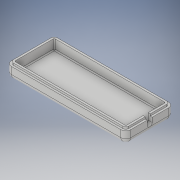
# Autodesk Inventor part: box_bottom
Saved by Autodesk Inventor 2017 (Build 210142000, 142)
## iProperties
Created: 2017-09-23
Part Number: box_bottom
Material: Generic
Document SubType Name: Modeling
Designer: Mitch
Density: 1 g/cm^3
Appearance: Default
Author: Mitch
Autodesk Inventor part; units mm, degrees
ref_plane "YZ Plane" through (0, 0, 0) normal (1, 0, 0) x (0, 1, 0)
ref_plane "XZ Plane" through (0, 0, 0) normal (0, 1, 0) x (-1, 0, 0)
ref_plane "XY Plane" through (0, 0, 0) normal (0, 0, 1) x (1, 0, 0)
sketch "Sketch1" plane through (0, 0, 0) normal (0, 1, 0) x (-1, 0, 0)
  line L0 (0, 0) -> (76.2, 0)
  line L1 (76.2, 0) -> (76.2, -30.48)
  line L2 (76.2, -30.48) -> (0, -30.48)
  line L3 (0, -30.48) -> (0, 0)
  dimension "d0" = 76.2
  dimension "d1" = 30.48
  constraints: 8 end point, 2 parallel, 1 horizontal, 1 perpendicular
  measures "d0" distance of L1.end L2.end
  measures "d1" distance of L0.end L1.end
extrude "Extrusion1" add sketch "Sketch1" along normal blind 8.89
fillet "Fillet1" radius 3.175 8 edges at (0, 4.445, 0) (0, 4.445, -30.48) (0, 0, -15.24) (-38.1, 0, 0) (-76.2, 4.445, 0) (-76.2, 0, -15.24) (-76.2, 4.445, -30.48) (-38.1, 0, -30.48)
shell "Shell1" thickness 2.54 removed faces 1 at (-26.4583, 8.89, -20.32)
sketch "Sketch2" plane through (0, 8.89, 0) normal (0, 1, 0) x (1, 0, 0)
  arc A0 (-76.2, 3.175) -> (-73.025, 0) centre (-73.025, 3.175) ccw projected
  line L0 (-76.2, 27.305) -> (-76.2, 3.175) projected
  arc A1 (-73.025, 30.48) -> (-76.2, 27.305) centre (-73.025, 27.305) ccw projected
  line L1 (-3.175, 30.48) -> (-73.025, 30.48) projected
  line L2 (-73.025, 0) -> (-3.175, 0) projected
  arc A2 (-3.175, 0) -> (0, 3.175) centre (-3.175, 3.175) ccw projected
  line L3 (0, 3.175) -> (0, 27.305) projected
  arc A3 (0, 27.305) -> (-3.175, 30.48) centre (-3.175, 27.305) ccw projected
  arc A4 (-73.025, 29.21) -> (-74.93, 27.305) centre (-73.025, 27.305) ccw
  line L4 (-74.93, 27.305) -> (-74.93, 3.175)
  arc A5 (-74.93, 3.175) -> (-73.025, 1.27) centre (-73.025, 3.175) ccw
  line L5 (-73.025, 1.27) -> (-3.175, 1.27)
  arc A6 (-3.175, 1.27) -> (-1.27, 3.175) centre (-3.175, 3.175) ccw
  line L6 (-1.27, 3.175) -> (-1.27, 27.305)
  arc A7 (-1.27, 27.305) -> (-3.175, 29.21) centre (-3.175, 27.305) ccw
  line L7 (-3.175, 29.21) -> (-73.025, 29.21)
  point P0 (0, 0)
  dimension "d6" = 1.27
  constraints: 8 end point, 8 point on circle, 4 centre point, 7 other
  measures "d6" distance between parallel lines of L1 L7
extrude "Extrusion2" cut sketch "Sketch2" against normal blind 1.27
sketch "Sketch3" plane through (0, 3.175, -3.175) normal (1, 0, 0) x (0, 0, -1)
  line L0 (0, 5.715) -> (24.13, 5.715) projected
  line L1 (12.065, 5.715) -> (12.065, 0.3712)
  line L2 (13.6525, 5.715) -> (13.6525, 1.5875)
  line L3 (10.4775, 5.715) -> (10.4775, 1.5875)
  line L4 (12.065, 0) -> (12.065, 0)
  arc A0 (10.4775, 1.5875) -> (12.065, 0) centre (12.065, 1.5875) ccw
  arc A1 (12.065, 0) -> (13.6525, 1.5875) centre (12.065, 1.5875) ccw
  line L5 (10.4775, 5.715) -> (13.6525, 5.715)
  point P0 (-3.175, -3.175)
  dimension "d9" = 1.5875
  dimension "d10" = 1.5875
  dimension "d11" = 5.715
  dimension "d12" = 1.5875
  constraints: 10 end point, 4 point on circle, 4 tangent, 2 centre point, 2 parallel, 1 collinear, 1 concentric, 1 horizontal, 1 midpoint, 1 vertical
  measures "d9" distance between parallel lines of L1 L2
  measures "d10" distance between parallel lines of L1 L3
  measures "d11" distance between parallel lines of L4 L0
  measures "d12" radius of A0
extrude "Extrusion3" cut sketch "Sketch3" against normal blind 2.54
body "Solid1"
